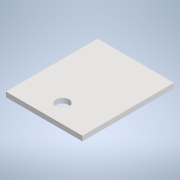
# Autodesk Inventor part: CLS_24.5N_plate
Saved by Autodesk Inventor 2021 (Build 250183000, 183)
## iProperties
Created: 2021-01-01
Part Number: CLS_24.5N_plate
Material: ステンレス鋼
Document SubType Name: Modeling
Designer: YusukeKunita
Density: 8 g/cm^3
Appearance: 半つや出し
Author: YusukeKunita
Autodesk Inventor part; units mm, degrees
ref_plane "YZ Plane" through (0, 0, 0) normal (1, 0, 0) x (0, 1, 0)
ref_plane "XZ Plane" through (0, 0, 0) normal (0, 1, 0) x (-1, 0, 0)
ref_plane "XY Plane" through (0, 0, 0) normal (0, 0, 1) x (1, 0, 0)
sketch "スケッチ1" plane through (0, 0, 0) normal (0, 0, 1) x (1, 0, 0)
  line L0 (0, 0) -> (25, 0)
  line L1 (25, 0) -> (25, 30)
  line L2 (25, 30) -> (0, 30)
  line L3 (0, 30) -> (0, 0)
  dimension "d0" = 25
  dimension "d1" = 30
  constraints: 8 end point, 2 parallel, 1 horizontal, 1 perpendicular
  measures "d0" distance of L0.start L0.end
  measures "d1" distance of L0.end L1.end
extrude "押し出し1" add sketch "スケッチ1" along normal blind 1.6
sketch "スケッチ2" plane through (0, 0, 1.6) normal (0, 0, 1) x (1, 0, 0)
  line L0 (0, 0) -> (25, 0) projected
  point P0 (12.5, 6)
  point P1 (12.5, 0)
  dimension "d4" = 6
  constraints: 1 midpoint, 1 vertical alignment
  measures "d4" distance from line of L0 point (12.5, 6)
hole "穴1" at (12.5, 6, 1.6) direction (0, 0, -1) diameter 4.2 end through all
